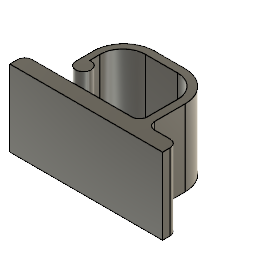
CableClip (Autodesk Fusion 360 design; units mm, degrees)
Autodesk Fusion 360 part; units mm, degrees
note: some values were not read from the file. Set by a fixed rule: which sketch regions a step uses.
sketch "Sketch1" plane through (0, 0, 0) normal (0, 0, 1) x (1, 0, 0)
  line L0 (4, 4.645) -> (4, 6.9613)
  line L1 (8, 10.9613) -> (12, 10.9613)
  line L2 (16, 6.9613) -> (16, 2.9855)
  line L3 (13, 2) -> (15, 2)
  line L4 (15, 2.9855) -> (15, 6.9613)
  line L5 (12, 9.9613) -> (7.8172, 9.9613)
  line L6 (17, 1.9855) -> (19, 1.9855)
  arc A0 (16, 2.9855) -> (17, 1.9855) centre (17, 2.9855) ccw
  line L7 (14, 1.9855) -> (1, 1.9855)
  arc A1 (14, 1.9855) -> (15, 2.9855) centre (14, 2.9855) ccw
  line L8 (0, 0.9855) -> (0, 0)
  line L9 (0, 0) -> (20, 0)
  line L10 (20, 0) -> (20, 0.9855)
  arc A2 (1, 1.9855) -> (0, 0.9855) centre (1, 0.9855) ccw
  arc A3 (20, 0.9855) -> (19, 1.9855) centre (19, 0.9855) ccw
  arc A4 (4, 4.645) -> (4.8517, 5.6339) centre (5, 4.645) ccw
  arc A5 (8, 10.9613) -> (4, 6.9613) centre (8, 6.9613) ccw
  arc A6 (16, 6.9613) -> (12, 10.9613) centre (12, 6.9613) ccw
  arc A7 (7.8172, 9.9613) -> (4.8173, 6.9821) centre (7.8172, 6.9613) ccw
  arc A8 (15, 6.9613) -> (12, 9.9613) centre (12, 6.9613) ccw
  line L11 (4.8173, 6.9821) -> (4.8517, 5.6339)
  dimension "d5" = 1
  dimension "d6" = 1
  dimension "d9" = 1
  dimension "d10" = 1
  dimension "d12" = 1
  dimension "d13" = 1
  dimension "d14" = 4
  dimension "d15" = 4
  dimension "d16" = 20
  dimension "d21" = 1
  dimension "d23" = 4
  dimension "d24" = 4
  dimension "d25" = 3
  dimension "d26" = 3
  measures "d5" radius of A0
  measures "d6" radius of A1
  measures "d9" radius of A2
  measures "d10" radius of A3
  measures "d12" distance of L1 L5
  measures "d13" distance of L2 L4
  measures "d14" distance of L0 L8
  measures "d15" distance of L2 L10
  measures "d16" distance of L8 L10
  measures "d21" radius of A4
  measures "d23" radius of A5
  measures "d24" radius of A6
  measures "d25" radius of A7
  measures "d26" radius of A8
extrude "Extrude1" add sketch "Sketch1" along normal blind 10
named bodies: "CableClip"
